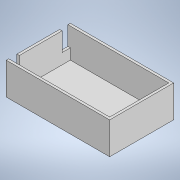
# Autodesk Inventor part: Крышка аккумулятора
Saved by Autodesk Inventor 2020 (Build 240168000, 168)
## iProperties
Created: 2021-08-09
Part Number: Крышка аккумулятора
Material: Типовые
Document SubType Name: Modeling
Designer: Антон
Density: 1 g/cm^3
Appearance: По умолчанию
Author: Антон
Autodesk Inventor part; units mm, degrees
ref_plane "YZ Plane" through (0, 0, 0) normal (1, 0, 0) x (0, 1, 0)
ref_plane "XZ Plane" through (0, 0, 0) normal (0, 1, 0) x (-1, 0, 0)
ref_plane "XY Plane" through (0, 0, 0) normal (0, 0, 1) x (1, 0, 0)
sketch "Эскиз1" plane through (0, 0, 0) normal (0, 1, 0) x (-1, 0, 0)
  line L0 (0, 0) -> (63.1, 0)
  line L1 (63.1, 0) -> (63.1, -39.1)
  line L2 (63.1, -39.1) -> (0, -39.1)
  line L3 (0, -39.1) -> (0, 0)
  dimension "d0" = 63.1
  dimension "d1" = 39.1
  constraints: 8 end point, 2 parallel, 1 horizontal, 1 perpendicular
  measures "d0" distance of L1.end L2.end
  measures "d1" distance of L0.end L1.end
extrude "Выдавливание1" add sketch "Эскиз1" along normal blind 19.5
shell "Оболочка1" thickness 1.5 removed faces 1 at (-42.0667, 19.5, -26.0667)
sketch "Эскиз2" plane through (0, 19.5, 0) normal (0, 1, 0) x (1, 0, 0)
  line L0 (-61.6, 37.6) -> (-61.6, 1.5) projected
  line L1 (-63.1, 39.1) -> (-63.1, 0) projected
  line L2 (-61.6, 37.6) -> (-63.1, 37.6)
  line L3 (-63.1, 37.6) -> (-63.1, 32.6)
  line L4 (-63.1, 32.6) -> (-61.6, 32.6)
  line L5 (-61.6, 32.6) -> (-61.6, 37.6)
  line L6 (-61.6, 1.5) -> (-63.1, 1.5)
  line L7 (-63.1, 1.5) -> (-63.1, 6.5)
  line L8 (-63.1, 6.5) -> (-61.6, 6.5)
  line L9 (-61.6, 6.5) -> (-61.6, 1.5)
  point P0 (0, 0)
  dimension "d5" = 5
  constraints: 16 end point, 5 parallel, 2 horizontal, 2 perpendicular, 1 collinear, 1 point on line
  measures "d5" distance of L3.end L2.end
extrude "Выдавливание2" cut sketch "Эскиз2" against normal blind 11.5 contours L0 L4 L1 L2 | L0 L6 L1 L8
